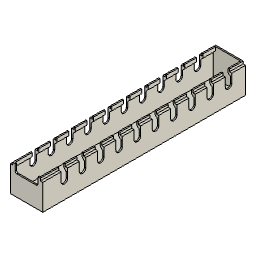
HarpejjiCover v1 (Autodesk Fusion 360 design; units mm, degrees)
Autodesk Fusion 360 part; units mm, degrees
note: some values were not read from the file. Set by a fixed rule: which face or edge a step refers to.
sketch "Schizzo1" plane through (0, 0, 0) normal (0, 1, 0) x (1, 0, 0)
  line L0 (0, 0) -> (40, 0)
  line L1 (40, 0) -> (40, -35)
  line L2 (40, -35) -> (0, -35)
  line L3 (0, -35) -> (0, 0)
  line L4 (3, -35) -> (3, -32)
  line L5 (3, -32) -> (0, -32)
  line L6 (37, -35) -> (37, -32)
  line L7 (37, -32) -> (40, -32)
  dimension "d1" = 3
  dimension "d2" = 40
  dimension "d3" = 35
  constraint horizontal L0
  constraint vertical L1
  constraint horizontal L2
  constraint vertical L3
  constraint coincident L0.start L3.end
  constraint coincident L2 L4.start
  constraint perpendicular L2 L4
  constraint coincident L3 L5.end
  constraint perpendicular L3 L5
  constraint coincident L2 L6.start
  constraint perpendicular L2 L6
  constraint coincident L1 L7.end
  constraint perpendicular L1 L7
  constraint equal L4 L5
  constraint equal L6 L7
  constraint equal L4 L6
  measures "d1" distance of L4.end L5.end
  measures "d2" distance of L1.end L2.end
  measures "d3" distance of L0.end L1.end
extrude "Estrusione1" add sketch "Schizzo1" along normal blind 250 contours L0 L1 L2 L3 L4 L5 L6 L7
shell "Svuotamento1" thickness 1.6 removed faces 1 at (25.6667, 83.3333, 35)
chamfer "Smusso1" distance 3 angle 45 2 edges at (38.4, 125, 30.4) (1.6, 125, 30.4)
sketch "Schizzo2" plane through (40, 0, 0) normal (1, 0, 0) x (0, 1, 0)
  line L0 (0, 32) -> (0, 0)
  line L1 (0, 0) -> (250, 0)
  line L2 (250, 0) -> (250, 32)
  line L3 (250, 32) -> (0, 32)
  line L4 (0, 35) -> (0, 32)
  line L5 (0, 32) -> (250, 32)
  line L6 (250, 32) -> (250, 35)
  line L7 (250, 35) -> (0, 35)
  line L8 (229, 35) -> (229, 17) construction
  line L9 (233, 35) -> (225, 35)
  line L10 (225, 35) -> (225, 17)
  line L11 (225, 17) -> (233, 17)
  line L12 (233, 17) -> (233, 35)
  dimension "d9" = 21
  dimension "d10" = 18
  dimension "d11" = 8
  constraint coincident L7 L8.start
  constraint perpendicular L5 L8
  constraint horizontal L9
  constraint vertical L10
  constraint horizontal L11
  constraint vertical L12
  constraint coincident L7 L9.start
  constraint midpoint L8.end L11
  measures "d9" distance of L2 L8
  measures "d10" distance of L9.start L11.end
  measures "d11" distance of L10.end L11.end
extrude "Estrusione2" cut sketch "Schizzo2" against normal blind 55 contours L3 L5 L7 L9 L10 L12 | L3 L5 L10 L11 L12
fillet "Raccordo1" radius 4 4 edges at (0.8, 225, 17) (0.8, 233, 17) (39.2, 225, 17) (39.2, 233, 17)
pattern_linear "Serie R1" count 10 spacing 22.5 along (0, -1, 0) of "Estrusione2", "Raccordo1"
sketch "Schizzo3" plane through (0, 0, 0) normal (0, -1, 0) x (1, 0, 0)
  line L0 (37, 32) -> (37, 35)
  line L1 (37, 35) -> (3, 35)
  line L2 (3, 35) -> (3, 32)
  line L3 (3, 32) -> (0, 32)
  line L4 (0, 32) -> (0, 0)
  line L5 (0, 0) -> (40, 0)
  line L6 (40, 0) -> (40, 32)
  line L7 (40, 32) -> (37, 32)
  line L8 (6, 35) -> (34, 35)
  line L9 (34, 35) -> (34, 25)
  line L10 (34, 25) -> (6, 25)
  line L11 (6, 25) -> (6, 35)
  line L12 (37, 32) -> (34, 32) construction
  line L13 (3, 32) -> (6, 32) construction
  dimension "d20" = 10
  dimension "d21" = 28
  constraint horizontal L8
  constraint vertical L9
  constraint horizontal L10
  constraint vertical L11
  constraint coincident L1 L8.start
  constraint coincident L0.start L7.end
  constraint coincident L9 L12.end
  constraint perpendicular L9 L12
  constraint coincident L2.end L3.start
  constraint coincident L11 L13.end
  constraint perpendicular L11 L13
  constraint equal L12 L13
  measures "d20" distance of L1 L10
  measures "d21" distance of L9 L11
extrude "Estrusione3" cut sketch "Schizzo3" against normal blind 11 contours L1 L8 L9 L10 L11
fillet "Raccordo2" radius 2 2 edges at (34, 0.8, 25) (6, 0.8, 25)
extrude "Estrusione4" cut 1 faces at (26.1333, 83.8667, 1.6) along direction (0, 0, -1) blind 0.8
